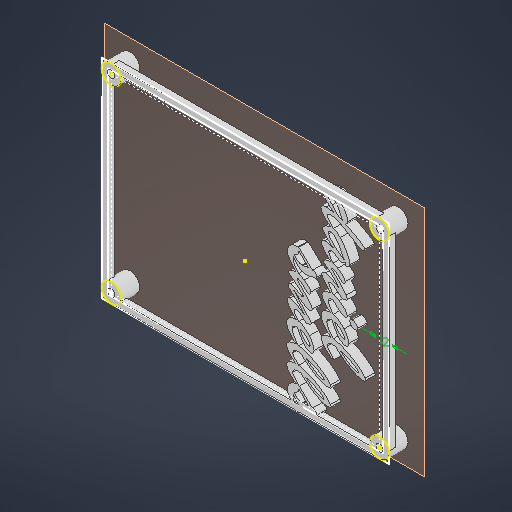
# Autodesk Inventor part: pcb standoff v1
Saved by Autodesk Inventor 2026.1 (Build 301233020, 233B)
## iProperties
Created: 2026-02-25
Part Number: pcb standoff v1
Material: Generic
Document SubType Name: Modeling
Designer: stoof
Density: 1 g/cm^3
Appearance: Default
Author: stoof
Autodesk Inventor part; units mm, degrees
ref_plane "YZ Plane" through (0, 0, 0) normal (1, 0, 0) x (0, 1, 0)
ref_plane "XZ Plane" through (0, 0, 0) normal (0, 1, 0) x (-1, 0, 0)
ref_plane "XY Plane" through (0, 0, 0) normal (0, 0, 1) x (1, 0, 0)
ref_plane "Work Plane1" through (0, 0, 0) normal (0, 0, 1) x (1, 0, 0)
sketch "Sketch1" plane through (0, 0, 0) normal (0, 0, 1) x (1, 0, 0)
  circle A0 centre (42.5, 30) radius 1.05 projected
  circle A1 centre (42.5, -30) radius 1.05 projected
  circle A2 centre (-42.5, -30) radius 1.05 projected
  circle A3 centre (-42.5, 30) radius 1.05 projected
  circle A4 centre (-42.5, 30) radius 3.05
  circle A5 centre (42.5, 30) radius 3.05
  circle A6 centre (42.5, -30) radius 3.05
  circle A7 centre (-42.5, -30) radius 3.05
  point P0 (0, 0)
  dimension "d0" = 2
  dimension "d1" = 2
  dimension "d2" = 2
  dimension "d3" = 2
  constraints: 4 centre point
  measures "d0" radial gap between concentric circles of A3 A4
  measures "d1" radial gap between concentric circles of A0 A5
  measures "d2" radial gap between concentric circles of A1 A6
  measures "d3" radial gap between concentric circles of A2 A7
extrude "Extrusion1" add sketch "Sketch1" along normal blind 6 contours A0 | A1 | A2 | A3 | A4 | A5 | A6 | A7
sketch "Sketch2" plane through (-42.5, 30, 6) normal (0, 0, 1) x (1, 0, 0)
  line L0 (85, 0) -> (0, 0) construction
  line L1 (0, 0) -> (0, -60) construction
  line L2 (0, -60) -> (85, -60) construction
  line L3 (85, -60) -> (85, 0) construction
  line L4 (86, 1) -> (-1, 1)
  line L5 (-1, 1) -> (-1, -61)
  line L6 (-1, -61) -> (86, -61)
  line L7 (86, -61) -> (86, 1)
  line L8 (88, 3) -> (-3, 3)
  line L9 (-3, 3) -> (-3, -63)
  line L10 (-3, -63) -> (88, -63)
  line L11 (88, -63) -> (88, 3)
  circle A0 centre (0, -60) radius 3.05 projected
  circle A1 centre (85, -60) radius 3.05 projected
  circle A2 centre (85, 0) radius 3.05 projected
  circle A3 centre (0, 0) radius 3.05 projected
  point P0 (42.5, -30)
  point P1 (85.55, -63)
  point P2 (88, -60.55)
  point P3 (88, 0.55)
  point P4 (85.55, 3)
  point P5 (-0.55, 3)
  point P6 (-3, 0.55)
  point P7 (-3, -60.55)
  point P8 (-0.55, -63)
  point P9 (88, -0.55)
  point P10 (86, -2.8814)
  point P11 (86, -57.1186)
  point P12 (88, -59.45)
  point P13 (0.55, 3)
  point P14 (2.8814, 1)
  point P15 (82.1186, 1)
  point P16 (84.45, 3)
  point P17 (84.45, -63)
  point P18 (82.1186, -61)
  point P19 (2.8814, -61)
  point P20 (0.55, -63)
  point P21 (-1, -2.8814)
  point P22 (-3, -0.55)
  point P23 (-3, -59.45)
  point P24 (-1, -57.1186)
  dimension "d6" = 1
  dimension "d7" = 2
  constraints: 24 end point, 6 parallel, 3 perpendicular, 1 horizontal, 6 other
  measures "d6" distance between parallel lines of L3 L7
  measures "d7" distance between parallel lines of L7 L11
extrude "Extrusion2" add sketch "Sketch2" against normal blind 2 contours L4 A3 L8 A2 | A2 L11 A1 L7 | A1 L10 A0 L6 | L5 A0 L9 A3
sketch "Sketch3" plane through (0, 0, 6) normal (0, 0, 1) x (1, 0, 0)
  line L0 (38.1473, 32.6739) -> (38.1473, 6.3376) construction
  line L1 (38.1473, 6.3376) -> (30.1508, 6.3376) construction
  line L2 (30.1508, 6.3376) -> (30.1508, 32.6739) construction
  line L3 (30.1508, 32.6739) -> (38.1473, 32.6739) construction
  line L4 (27.1524, 12.2976) -> (27.1524, -13.1616) construction
  line L5 (27.1524, -13.1616) -> (19.2192, -13.1616) construction
  line L6 (19.2192, -13.1616) -> (19.2192, 12.2976) construction
  line L7 (19.2192, 12.2976) -> (27.1524, 12.2976) construction
  line L8 (16.645, 12.1571) -> (16.9259, 12.1571)
  spline S0 degree 2 poles (16.9259, 12.1571) (20.0444, 9.1931) (21.2947, 8.0834) knots 0 0 0 1 1 1
  spline S1 degree 2 poles (21.2947, 8.0834) (22.6994, 7.8305) (22.6994, 6.8753) knots 0 0 0 1 1 1
  spline S2 degree 2 poles (22.6994, 6.8753) (22.6994, 6.6365) (22.5589, 6.3555) knots 0 0 0 1 1 1
  line L9 (22.5589, 6.3555) -> (22.3482, 6.2853)
  spline S3 degree 2 poles (22.3482, 6.2853) (22.2077, 6.3415) (21.9549, 6.3415) knots 0 0 0 1 1 1
  spline S4 degree 2 poles (21.9549, 6.3415) (21.7301, 6.3415) (20.5501, 6.0044) (19.7494, 5.8217) (19.2437, 5.8217) knots 0 0 0 1 2 3 3 3
  spline S5 degree 2 poles (19.2437, 5.8217) (18.4992, 5.8217) (17.1085, 6.5101) (15.8302, 7.8165) (15.17, 8.8419) knots 0 0 0 1 2 3 3 3
  spline S6 degree 2 poles (15.17, 8.8419) (15.0998, 8.4346) (15.0998, 8.1958) knots 0 0 0 1 1 1
  spline S7 degree 2 poles (15.0998, 8.1958) (15.0998, 7.7181) (15.5633, 6.6365) (16.364, 5.4987) (16.9962, 4.7401) knots 0 0 0 1 2 3 3 3
  line L10 (16.9962, 4.7401) -> (16.2235, 4.7401)
  spline S8 degree 2 poles (16.2235, 4.7401) (14.7907, 6.2151) (13.3157, 8.5188) (13.3157, 9.3617) knots 0 0 0 1 2 2 2
  spline S9 degree 2 poles (13.3157, 9.3617) (13.3157, 10.4433) (14.2288, 11.3564) knots 0 0 0 1 1 1
  spline S10 degree 2 poles (14.2288, 11.3564) (14.7767, 11.8902) (15.7881, 12.1571) (16.645, 12.1571) knots 0 0 0 1 2 2 2
  line L11 (18.4009, 7.8867) -> (20.0725, 8.0834)
  spline S11 degree 2 poles (20.0725, 8.0834) (19.2718, 8.7998) (16.9962, 11.1176) knots 0 0 0 1 1 1
  spline S12 degree 2 poles (16.9962, 11.1176) (16.8416, 10.4293) (16.3359, 9.9376) (15.6195, 9.4741) knots 0 0 0 1 2 2 2
  spline S13 degree 2 poles (15.6195, 9.4741) (15.9426, 8.7015) (17.0523, 7.8586) (18.0076, 7.8586) knots 0 0 0 1 2 2 2
  spline S14 degree 2 poles (18.0076, 7.8586) (18.1199, 7.8586) (18.3026, 7.8727) (18.4009, 7.8867) knots 0 0 0 1 2 2 2
  spline S15 degree 2 poles (15.3947, -0.4434) (16.7995, -2.0308) (18.8645, -4.2924) (20.0585, -5.5848) (20.8873, -6.5681) (20.8873, -6.7085) knots 0 0 0 1 2 3 4 4 4
  spline S16 degree 2 poles (20.8873, -6.7085) (20.8873, -6.9754) (19.7775, -7.4531) (19.4544, -7.4531) knots 0 0 0 1 2 2 2
  spline S17 degree 2 poles (19.4544, -7.4531) (19.2297, -7.4531) (17.6142, -5.9921) (16.659, -5.2757) (16.1393, -5.2757) knots 0 0 0 1 2 3 3 3
  spline S18 degree 2 poles (16.1393, -5.2757) (15.8302, -5.2757) (15.4509, -5.6831) (15.4509, -5.9781) knots 0 0 0 1 2 2 2
  spline S19 degree 2 poles (15.4509, -5.9781) (15.4509, -6.3012) (16.1393, -7.2283) (17.0102, -8.2257) knots 0 0 0 1 2 2 2
  line L12 (17.0102, -8.2257) -> (16.2095, -8.2257)
  spline S20 degree 2 poles (16.2095, -8.2257) (15.2683, -7.2423) (13.8917, -5.6128) (13.2174, -4.4048) (13.2174, -4.0114) knots 0 0 0 1 2 3 3 3
  spline S21 degree 2 poles (13.2174, -4.0114) (13.2174, -3.6462) (13.7652, -3.1686) (14.1586, -3.1686) knots 0 0 0 1 2 2 2
  spline S22 degree 2 poles (14.1586, -3.1686) (14.5519, -3.1686) (15.3526, -3.4495) (16.4483, -4.0114) (17.9935, -4.9526) (18.6397, -5.3459) knots 0 0 0 1 2 3 4 4 4
  spline S23 degree 2 poles (18.6397, -5.3459) (17.6845, -4.18) (15.9285, -2.3679) (14.6081, -1.216) (14.2288, -0.8929) knots 0 0 0 1 2 3 3 3
  spline S24 degree 2 poles (14.2288, -0.8929) (13.5124, -0.2467) (13.5124, 0.3011) knots 0 0 0 1 1 1
  spline S25 degree 2 poles (13.5124, 0.3011) (13.5124, 0.8911) (14.3693, 0.8911) knots 0 0 0 1 1 1
  spline S26 degree 2 poles (14.3693, 0.8911) (14.7064, 0.8911) (16.4904, 0.0061) (17.853, -0.8227) knots 0 0 0 1 2 2 2
  spline S27 degree 2 poles (17.853, -0.8227) (17.9514, -0.8929) (18.148, -0.8929) knots 0 0 0 1 1 1
  spline S28 degree 2 poles (18.148, -0.8929) (18.3728, -0.8929) (18.3728, -0.6541) knots 0 0 0 1 1 1
  spline S29 degree 2 poles (18.3728, -0.6541) (18.3728, -0.4153) (17.4176, 0.5399) (15.9145, 1.9025) knots 0 0 0 1 2 2 2
  spline S30 degree 2 poles (15.9145, 1.9025) (15.4931, 2.2818) (14.1305, 3.237) (13.6669, 3.6444) (13.6669, 3.8551) knots 0 0 0 1 2 3 3 3
  spline S31 degree 2 poles (13.6669, 3.8551) (13.6669, 4.2625) (15.1278, 4.9789) (16.1112, 4.9789) knots 0 0 0 1 2 2 2
  spline S32 degree 2 poles (16.1112, 4.9789) (16.8135, 4.9789) (17.853, 4.5153) (18.6116, 4.0237) knots 0 0 0 1 2 2 2
  spline S33 degree 2 poles (18.6116, 4.0237) (19.7213, 3.2511) (20.6766, 2.2677) (20.6766, 1.7339) knots 0 0 0 1 2 2 2
  spline S34 degree 2 poles (20.6766, 1.7339) (20.6766, 1.3968) (20.4097, 0.9332) (20.1849, 0.9332) knots 0 0 0 1 2 2 2
  spline S35 degree 2 poles (20.1849, 0.9332) (19.9461, 0.9332) (18.8364, 1.7761) (18.2604, 2.4223) knots 0 0 0 1 2 2 2
  spline S36 degree 2 poles (18.2604, 2.4223) (17.9233, 2.7735) (16.954, 3.3915) (16.7433, 3.3915) knots 0 0 0 1 2 2 2
  spline S37 degree 2 poles (16.7433, 3.3915) (16.4343, 3.3915) (16.4343, 3.1527) knots 0 0 0 1 1 1
  spline S38 degree 2 poles (16.4343, 3.1527) (16.4343, 2.9561) (18.0357, 1.3687) (19.918, -0.5136) (21.1682, -2.1431) (21.1682, -2.705) knots 0 0 0 1 2 3 4 4 4
  spline S39 degree 2 poles (21.1682, -2.705) (21.1682, -3.0422) (20.6485, -3.4917) (20.2692, -3.4917) knots 0 0 0 1 2 2 2
  spline S40 degree 2 poles (20.2692, -3.4917) (20.0304, -3.4917) (18.7099, -2.8034) (16.7714, -1.4829) (15.3947, -0.4434) knots 0 0 0 1 2 3 3 3
  line L13 (16.5466, -9.9816) -> (16.2657, -9.9816)
  spline S41 degree 2 poles (16.2657, -9.9816) (15.5914, -9.9816) (14.8328, -10.6418) (14.8328, -11.1756) knots 0 0 0 1 2 2 2
  spline S42 degree 2 poles (14.8328, -11.1756) (14.8328, -11.7375) (15.3667, -12.9456) (16.2235, -14.1256) (16.9681, -14.9825) knots 0 0 0 1 2 3 3 3
  line L14 (16.9681, -14.9825) -> (16.2657, -14.9825)
  spline S43 degree 2 poles (16.2657, -14.9825) (14.7064, -13.6901) (13.0488, -11.4285) (13.0488, -10.2625) knots 0 0 0 1 2 2 2
  spline S44 degree 2 poles (13.0488, -10.2625) (13.0488, -9.2511) (14.6362, -8.0571) (15.9988, -8.0571) knots 0 0 0 1 2 2 2
  spline S45 degree 2 poles (15.9988, -8.0571) (17.2069, -8.0571) (19.1735, -9.1809) (20.2551, -10.4452) knots 0 0 0 1 2 2 2
  spline S46 degree 2 poles (20.2551, -10.4452) (20.9997, -11.3161) (21.7582, -13.0299) (21.7582, -13.7042) knots 0 0 0 1 2 2 2
  spline S47 degree 2 poles (21.7582, -13.7042) (21.7582, -14.238) (21.2666, -14.8701) (20.7749, -14.8701) knots 0 0 0 1 2 2 2
  spline S48 degree 2 poles (20.7749, -14.8701) (20.0444, -14.8701) (18.6116, -13.8025) (17.2069, -11.597) (16.5466, -9.9816) knots 0 0 0 1 2 3 3 3
  spline S49 degree 2 poles (17.2911, -10.094) (17.6985, -11.1194) (18.8926, -12.5804) (19.9742, -13.2827) (20.2271, -13.2827) knots 0 0 0 1 2 3 3 3
  spline S50 degree 2 poles (20.2271, -13.2827) (20.494, -13.2827) (20.494, -13.0439) knots 0 0 0 1 1 1
  spline S51 degree 2 poles (20.494, -13.0439) (20.494, -12.8332) (19.9602, -11.9061) (19.1173, -10.9649) (17.9795, -10.2064) (17.2911, -10.094) knots 0 0 0 1 2 3 4 4 4
  line L15 (17.0945, -20.475) -> (16.2516, -20.475)
  spline S52 degree 2 poles (16.2516, -20.475) (13.0769, -18.0729) (13.0769, -16.5698) knots 0 0 0 1 1 1
  spline S53 degree 2 poles (13.0769, -16.5698) (13.0769, -15.7551) (14.8469, -14.8279) (16.2938, -14.8279) knots 0 0 0 1 2 2 2
  spline S54 degree 2 poles (16.2938, -14.8279) (17.4597, -14.8279) (20.6766, -15.9236) (23.9918, -17.7779) (26.4501, -19.7726) (26.9417, -20.6155) knots 0 0 0 1 2 3 4 4 4
  spline S55 degree 2 poles (26.9417, -20.6155) (27.1524, -20.9667) (27.1524, -21.1493) knots 0 0 0 1 1 1
  spline S56 degree 2 poles (27.1524, -21.1493) (27.1524, -21.4021) (26.731, -21.5567) (26.2113, -21.5567) knots 0 0 0 1 2 2 2
  spline S57 degree 2 poles (26.2113, -21.5567) (24.6239, -21.5567) (19.9882, -18.9579) (17.5721, -16.6401) knots 0 0 0 1 2 2 2
  spline S58 degree 2 poles (17.5721, -16.6401) (16.9681, -16.5277) (16.645, -16.5277) knots 0 0 0 1 1 1
  spline S59 degree 2 poles (16.645, -16.5277) (15.9145, -16.5277) (15.0014, -17.1598) (15.0014, -17.7217) knots 0 0 0 1 2 2 2
  spline S60 degree 2 poles (15.0014, -17.7217) (15.0014, -18.0027) (15.4509, -18.6769) (16.1112, -19.4074) (17.0945, -20.475) knots 0 0 0 1 2 3 3 3
  spline S61 degree 2 poles (19.1595, -17.0474) (19.7494, -17.6374) (21.2385, -18.7612) (22.9382, -19.7445) (24.2868, -20.3064) (24.6239, -20.3064) knots 0 0 0 1 2 3 4 4 4
  spline S62 degree 2 poles (24.6239, -20.3064) (24.8908, -20.3064) (24.8908, -20.1238) knots 0 0 0 1 1 1
  spline S63 degree 2 poles (24.8908, -20.1238) (24.8908, -20.0536) (24.7644, -19.8569) knots 0 0 0 1 1 1
  spline S64 degree 2 poles (24.7644, -19.8569) (24.1884, -19.1546) (20.8592, -17.4127) (19.1595, -17.0474) knots 0 0 0 1 2 2 2
  line L16 (17.0945, -25.8411) -> (16.2516, -25.8411)
  spline S65 degree 2 poles (16.2516, -25.8411) (13.0769, -23.439) (13.0769, -21.9359) knots 0 0 0 1 1 1
  spline S66 degree 2 poles (13.0769, -21.9359) (13.0769, -21.1212) (14.8469, -20.1941) (16.2938, -20.1941) knots 0 0 0 1 2 2 2
  spline S67 degree 2 poles (16.2938, -20.1941) (17.4597, -20.1941) (20.6766, -21.2898) (23.9918, -23.144) (26.4501, -25.1387) (26.9417, -25.9816) knots 0 0 0 1 2 3 4 4 4
  spline S68 degree 2 poles (26.9417, -25.9816) (27.1524, -26.3328) (27.1524, -26.5154) knots 0 0 0 1 1 1
  spline S69 degree 2 poles (27.1524, -26.5154) (27.1524, -26.7682) (26.731, -26.9228) (26.2113, -26.9228) knots 0 0 0 1 2 2 2
  spline S70 degree 2 poles (26.2113, -26.9228) (24.6239, -26.9228) (19.9882, -24.324) (17.5721, -22.0062) knots 0 0 0 1 2 2 2
  spline S71 degree 2 poles (17.5721, -22.0062) (16.9681, -21.8938) (16.645, -21.8938) knots 0 0 0 1 1 1
  spline S72 degree 2 poles (16.645, -21.8938) (15.9145, -21.8938) (15.0014, -22.5259) (15.0014, -23.0878) knots 0 0 0 1 2 2 2
  spline S73 degree 2 poles (15.0014, -23.0878) (15.0014, -23.3688) (15.4509, -24.0431) (16.1112, -24.7735) (17.0945, -25.8411) knots 0 0 0 1 2 3 3 3
  spline S74 degree 2 poles (19.1595, -22.4136) (19.7494, -23.0035) (21.2385, -24.1273) (22.9382, -25.1107) (24.2868, -25.6726) (24.6239, -25.6726) knots 0 0 0 1 2 3 4 4 4
  spline S75 degree 2 poles (24.6239, -25.6726) (24.8908, -25.6726) (24.8908, -25.4899) knots 0 0 0 1 1 1
  spline S76 degree 2 poles (24.8908, -25.4899) (24.8908, -25.4197) (24.7644, -25.223) knots 0 0 0 1 1 1
  spline S77 degree 2 poles (24.7644, -25.223) (24.1884, -24.5207) (20.8592, -22.7788) (19.1595, -22.4136) knots 0 0 0 1 2 2 2
  line L17 (16.645, -25.6866) -> (16.9259, -25.6866)
  spline S78 degree 2 poles (16.9259, -25.6866) (20.0444, -28.6506) (21.2947, -29.7603) knots 0 0 0 1 1 1
  spline S79 degree 2 poles (21.2947, -29.7603) (22.6994, -30.0132) (22.6994, -30.9684) knots 0 0 0 1 1 1
  spline S80 degree 2 poles (22.6994, -30.9684) (22.6994, -31.2072) (22.5589, -31.4882) knots 0 0 0 1 1 1
  line L18 (22.5589, -31.4882) -> (22.3482, -31.5584)
  spline S81 degree 2 poles (22.3482, -31.5584) (22.2077, -31.5022) (21.9549, -31.5022) knots 0 0 0 1 1 1
  spline S82 degree 2 poles (21.9549, -31.5022) (21.7301, -31.5022) (20.5501, -31.8394) (19.7494, -32.022) (19.2437, -32.022) knots 0 0 0 1 2 3 3 3
  spline S83 degree 2 poles (19.2437, -32.022) (18.4992, -32.022) (17.1085, -31.3337) (15.8302, -30.0272) (15.17, -29.0018) knots 0 0 0 1 2 3 3 3
  spline S84 degree 2 poles (15.17, -29.0018) (15.0998, -29.4092) (15.0998, -29.648) knots 0 0 0 1 1 1
  spline S85 degree 2 poles (15.0998, -29.648) (15.0998, -30.1256) (15.5633, -31.2072) (16.364, -32.3451) (16.9962, -33.1036) knots 0 0 0 1 2 3 3 3
  line L19 (16.9962, -33.1036) -> (16.2235, -33.1036)
  spline S86 degree 2 poles (16.2235, -33.1036) (14.7907, -31.6287) (13.3157, -29.3249) (13.3157, -28.482) knots 0 0 0 1 2 2 2
  spline S87 degree 2 poles (13.3157, -28.482) (13.3157, -27.4004) (14.2288, -26.4873) knots 0 0 0 1 1 1
  spline S88 degree 2 poles (14.2288, -26.4873) (14.7767, -25.9535) (15.7881, -25.6866) (16.645, -25.6866) knots 0 0 0 1 2 2 2
  line L20 (18.4009, -29.957) -> (20.0725, -29.7603)
  spline S89 degree 2 poles (20.0725, -29.7603) (19.2718, -29.0439) (16.9962, -26.7261) knots 0 0 0 1 1 1
  spline S90 degree 2 poles (16.9962, -26.7261) (16.8416, -27.4144) (16.3359, -27.9061) (15.6195, -28.3697) knots 0 0 0 1 2 2 2
  spline S91 degree 2 poles (15.6195, -28.3697) (15.9426, -29.1423) (17.0523, -29.9851) (18.0076, -29.9851) knots 0 0 0 1 2 2 2
  spline S92 degree 2 poles (18.0076, -29.9851) (18.1199, -29.9851) (18.3026, -29.9711) (18.4009, -29.957) knots 0 0 0 1 2 2 2
  spline S93 degree 2 poles (27.9348, 27.2516) (26.7829, 28.263) (25.1815, 29.8503) (24.3948, 30.8477) (24.3948, 31.0303) knots 0 0 0 1 2 3 3 3
  spline S94 degree 2 poles (24.3948, 31.0303) (24.3948, 31.3394) (25.3641, 32.0839) (26.8531, 32.6036) (27.6117, 32.6036) knots 0 0 0 1 2 3 3 3
  spline S95 degree 2 poles (27.6117, 32.6036) (28.7214, 32.6036) (30.9831, 30.4544) (32.4721, 27.7011) (32.4721, 27.0128) knots 0 0 0 1 2 3 3 3
  spline S96 degree 2 poles (32.4721, 27.0128) (32.4721, 26.4509) (31.7697, 25.9171) knots 0 0 0 1 1 1
  spline S97 degree 2 poles (31.7697, 25.9171) (33.6099, 25.0321) (36.4756, 23.4447) (37.8663, 22.3631) (37.8663, 22.1383) knots 0 0 0 1 2 3 3 3
  spline S98 degree 2 poles (37.8663, 22.1383) (37.8663, 21.8855) (37.3746, 21.464) (37.0656, 21.464) knots 0 0 0 1 2 2 2
  spline S99 degree 2 poles (37.0656, 21.464) (36.4756, 21.464) (33.5678, 23.2059) (30.8145, 24.9057) (28.1455, 26.1137) (27.0217, 26.1137) knots 0 0 0 1 2 3 4 4 4
  spline S100 degree 2 poles (27.0217, 26.1137) (25.9822, 26.1137) (25.9822, 25.4535) knots 0 0 0 1 1 1
  spline S101 degree 2 poles (25.9822, 25.4535) (25.9822, 25.0461) (26.8953, 23.8381) (27.9629, 22.7143) knots 0 0 0 1 2 2 2
  line L21 (27.9629, 22.7143) -> (27.12, 22.7143)
  spline S102 degree 2 poles (27.12, 22.7143) (23.9313, 25.1866) (23.9313, 26.5211) knots 0 0 0 1 1 1
  spline S103 degree 2 poles (23.9313, 26.5211) (23.9313, 27.069) (24.746, 27.5325) (25.5608, 27.5325) knots 0 0 0 1 2 2 2
  spline S104 degree 2 poles (25.5608, 27.5325) (26.6565, 27.5325) (27.9348, 27.2516) knots 0 0 0 1 1 1
  spline S105 degree 2 poles (30.7302, 26.4087) (30.3931, 27.4342) (28.8619, 30.1734) (28.581, 30.4544) knots 0 0 0 1 2 2 2
  spline S106 degree 2 poles (28.581, 30.4544) (28.3422, 30.7072) (27.0919, 31.1006) (26.7689, 31.1006) knots 0 0 0 1 2 2 2
  spline S107 degree 2 poles (26.7689, 31.1006) (26.5722, 31.1006) (26.3193, 30.8758) (26.3193, 30.6932) knots 0 0 0 1 2 2 2
  spline S108 degree 2 poles (26.3193, 30.6932) (26.3193, 30.5387) (26.6003, 30.1313) (27.401, 29.2182) (27.5134, 29.0918) knots 0 0 0 1 2 3 3 3
  spline S109 degree 2 poles (27.5134, 29.0918) (27.6819, 28.8951) (28.8198, 27.5606) (29.4519, 26.9425) (30.2526, 26.5071) (30.7302, 26.4087) knots 0 0 0 1 2 3 4 4 4
  spline S110 degree 2 poles (30.0138, 21.3657) (31.6012, 19.6238) (33.1323, 16.3508) (33.1323, 15.4658) knots 0 0 0 1 2 2 2
  spline S111 degree 2 poles (33.1323, 15.4658) (33.1323, 15.227) (32.725, 14.8056) (32.2052, 14.5668) (32.0788, 14.5668) knots 0 0 0 1 2 3 3 3
  spline S112 degree 2 poles (32.0788, 14.5668) (31.8681, 14.5668) (31.6714, 14.8899) (31.545, 15.2972) knots 0 0 0 1 2 2 2
  spline S113 degree 2 poles (31.545, 15.2972) (31.3624, 15.2129) (30.7864, 14.9601) (30.4212, 14.8196) (30.2948, 14.8196) knots 0 0 0 1 2 3 3 3
  spline S114 degree 2 poles (30.2948, 14.8196) (30.0138, 14.8196) (28.5107, 15.9294) (27.8084, 16.3789) (27.2886, 16.3789) knots 0 0 0 1 2 3 3 3
  spline S115 degree 2 poles (27.2886, 16.3789) (26.4458, 16.3789) (26.4458, 15.6063) knots 0 0 0 1 1 1
  spline S116 degree 2 poles (26.4458, 15.6063) (26.4458, 14.7915) (27.9348, 13.0918) knots 0 0 0 1 1 1
  line L22 (27.9348, 13.0918) -> (27.2465, 13.0918)
  spline S117 degree 2 poles (27.2465, 13.0918) (24.0296, 15.9855) (24.0296, 17.2358) knots 0 0 0 1 1 1
  spline S118 degree 2 poles (24.0296, 17.2358) (24.0296, 17.6853) (24.6056, 18.0646) (25.1815, 18.0646) knots 0 0 0 1 2 2 2
  spline S119 degree 2 poles (25.1815, 18.0646) (26.0805, 18.0646) (27.8084, 17.4043) knots 0 0 0 1 1 1
  spline S120 degree 2 poles (27.8084, 17.4043) (25.9541, 19.076) (24.3808, 20.7055) (24.3808, 21.2393) knots 0 0 0 1 2 2 2
  spline S121 degree 2 poles (24.3808, 21.2393) (24.3808, 21.4921) (25.2517, 22.2366) (26.6424, 22.8266) (27.3869, 22.8266) knots 0 0 0 1 2 3 3 3
  spline S122 degree 2 poles (27.3869, 22.8266) (27.9207, 22.8266) (28.6372, 22.6159) (29.3957, 22.0259) (30.0138, 21.3657) knots 0 0 0 1 2 3 3 3
  spline S123 degree 2 poles (31.2781, 15.8872) (29.9155, 18.8653) (28.005, 21.3938) (27.0077, 21.3938) knots 0 0 0 1 2 2 2
  spline S124 degree 2 poles (27.0077, 21.3938) (26.6284, 21.3938) (26.1648, 21.1409) (26.1648, 20.9302) knots 0 0 0 1 2 2 2
  spline S125 degree 2 poles (26.1648, 20.9302) (26.1648, 20.8038) (26.3193, 20.4807) knots 0 0 0 1 1 1
  spline S126 degree 2 poles (26.3193, 20.4807) (27.0358, 19.2726) (29.3114, 17.2779) (31.2781, 15.8872) knots 0 0 0 1 2 2 2
  spline S127 degree 2 poles (30.0279, 5.464) (27.7803, 7.4869) (26.9093, 7.4869) knots 0 0 0 1 1 1
  spline S128 degree 2 poles (26.9093, 7.4869) (26.4177, 7.4869) (26.4177, 7.0795) knots 0 0 0 1 1 1
  spline S129 degree 2 poles (26.4177, 7.0795) (26.4177, 6.7564) (27.106, 5.6888) (28.005, 4.551) knots 0 0 0 1 2 2 2
  line L23 (28.005, 4.551) -> (27.2184, 4.551)
  spline S130 degree 2 poles (27.2184, 4.551) (25.617, 6.1805) (24.1982, 7.9223) (24.1982, 8.4702) knots 0 0 0 1 2 2 2
  spline S131 degree 2 poles (24.1982, 8.4702) (24.1982, 9.4114) (25.4343, 9.4114) knots 0 0 0 1 1 1
  spline S132 degree 2 poles (25.4343, 9.4114) (25.7996, 9.4114) (26.502, 9.1866) (27.2746, 8.7792) (28.7074, 7.9504) (29.6064, 7.4166) knots 0 0 0 1 2 3 4 4 4
  spline S133 degree 2 poles (29.6064, 7.4166) (29.2693, 8.0769) (28.286, 9.0602) knots 0 0 0 1 1 1
  spline S134 degree 2 poles (28.286, 9.0602) (27.6679, 9.6923) (26.5581, 10.5913) (25.1955, 11.6028) (24.732, 12.0804) (24.732, 12.3192) knots 0 0 0 1 2 3 4 4 4
  spline S135 degree 2 poles (24.732, 12.3192) (24.732, 12.6844) (26.2631, 13.3025) (27.2886, 13.3025) knots 0 0 0 1 2 2 2
  spline S136 degree 2 poles (27.2886, 13.3025) (27.9067, 13.3025) (28.6231, 13.0215) (29.2693, 12.5861) knots 0 0 0 1 2 2 2
  spline S137 degree 2 poles (29.2693, 12.5861) (30.4914, 11.7994) (31.6152, 10.6616) (31.6152, 10.1278) knots 0 0 0 1 2 2 2
  spline S138 degree 2 poles (31.6152, 10.1278) (31.6152, 9.7625) (31.3624, 9.313) (31.1095, 9.313) knots 0 0 0 1 2 2 2
  spline S139 degree 2 poles (31.1095, 9.313) (30.9971, 9.313) (30.7443, 9.4535) (30.5336, 9.6221) (30.2386, 9.903) knots 0 0 0 1 2 3 3 3
  spline S140 degree 2 poles (30.2386, 9.903) (28.2298, 11.7151) (27.6398, 11.7151) knots 0 0 0 1 1 1
  spline S141 degree 2 poles (27.6398, 11.7151) (27.3027, 11.7151) (27.3027, 11.4904) knots 0 0 0 1 1 1
  spline S142 degree 2 poles (27.3027, 11.4904) (27.3027, 11.364) (28.1876, 10.5632) (29.6205, 9.313) (31.1797, 7.6133) (31.8962, 6.5176) knots 0 0 0 1 2 3 4 4 4
  spline S143 degree 2 poles (31.8962, 6.5176) (32.3176, 5.9136) (32.3176, 5.5062) knots 0 0 0 1 1 1
  spline S144 degree 2 poles (32.3176, 5.5062) (32.3176, 5.3236) (31.3062, 4.9724) (30.8005, 4.9724) knots 0 0 0 1 2 2 2
  spline S145 degree 2 poles (30.8005, 4.9724) (30.5476, 4.9724) (30.0279, 5.464) knots 0 0 0 1 1 1
  line L24 (27.9629, -0.8432) -> (27.1341, -0.8432)
  spline S146 degree 2 poles (27.1341, -0.8432) (25.7012, 0.2665) (24.2403, 2.1769) (24.2403, 2.8512) knots 0 0 0 1 2 2 2
  spline S147 degree 2 poles (24.2403, 2.8512) (24.2403, 3.7924) (26.207, 4.7055) (27.3729, 4.7055) knots 0 0 0 1 2 2 2
  spline S148 degree 2 poles (27.3729, 4.7055) (27.8224, 4.7055) (28.6372, 4.5229) (29.171, 4.27) (29.7188, 3.9329) knots 0 0 0 1 2 3 3 3
  spline S149 degree 2 poles (29.7188, 3.9329) (32.2614, 2.3034) (32.2614, 0.9548) knots 0 0 0 1 1 1
  spline S150 degree 2 poles (32.2614, 0.9548) (32.2614, 0.2665) (31.7276, 0.2665) knots 0 0 0 1 1 1
  spline S151 degree 2 poles (31.7276, 0.2665) (31.3483, 0.2665) (29.789, 1.1655) (29.466, 1.5167) knots 0 0 0 1 2 2 2
  spline S152 degree 2 poles (29.466, 1.5167) (28.4967, 2.5141) (27.7522, 3.1181) (27.2605, 3.1181) knots 0 0 0 1 2 2 2
  spline S153 degree 2 poles (27.2605, 3.1181) (26.8531, 3.1181) (26.3053, 2.5) (26.3053, 2.0084) knots 0 0 0 1 2 2 2
  spline S154 degree 2 poles (26.3053, 2.0084) (26.3053, 1.4746) (27.0919, 0.1822) (27.9629, -0.8432) knots 0 0 0 1 2 2 2
  spline S155 degree 2 poles (33.0761, -0.0706) (33.0761, 0.2103) (33.5116, 0.7301) (33.8487, 0.7301) knots 0 0 0 1 2 2 2
  spline S156 degree 2 poles (33.8487, 0.7301) (34.3545, 0.7301) (35.5906, -0.2252) (35.5906, -0.7449) knots 0 0 0 1 2 2 2
  spline S157 degree 2 poles (35.5906, -0.7449) (35.5906, -1.0821) (35.1692, -1.5456) (34.7618, -1.5456) knots 0 0 0 1 2 2 2
  spline S158 degree 2 poles (34.7618, -1.5456) (34.2702, -1.5456) (33.0761, -0.6044) (33.0761, -0.0706) knots 0 0 0 1 2 2 2
  line L25 (27.5415, -2.5851) -> (27.2605, -2.5851)
  spline S159 degree 2 poles (27.2605, -2.5851) (26.5862, -2.5851) (25.8277, -3.2454) (25.8277, -3.7792) knots 0 0 0 1 2 2 2
  spline S160 degree 2 poles (25.8277, -3.7792) (25.8277, -4.3411) (26.3615, -5.5491) (27.2184, -6.7291) (27.9629, -7.586) knots 0 0 0 1 2 3 3 3
  line L26 (27.9629, -7.586) -> (27.2605, -7.586)
  spline S161 degree 2 poles (27.2605, -7.586) (25.7012, -6.2936) (24.0437, -4.032) (24.0437, -2.8661) knots 0 0 0 1 2 2 2
  spline S162 degree 2 poles (24.0437, -2.8661) (24.0437, -1.8547) (25.631, -0.6606) (26.9936, -0.6606) knots 0 0 0 1 2 2 2
  spline S163 degree 2 poles (26.9936, -0.6606) (28.2017, -0.6606) (30.1683, -1.7844) (31.25, -3.0487) knots 0 0 0 1 2 2 2
  spline S164 degree 2 poles (31.25, -3.0487) (31.9945, -3.9196) (32.753, -5.6334) (32.753, -6.3077) knots 0 0 0 1 2 2 2
  spline S165 degree 2 poles (32.753, -6.3077) (32.753, -6.8415) (32.2614, -7.4736) (31.7697, -7.4736) knots 0 0 0 1 2 2 2
  spline S166 degree 2 poles (31.7697, -7.4736) (31.0393, -7.4736) (29.6064, -6.406) (28.2017, -4.2006) (27.5415, -2.5851) knots 0 0 0 1 2 3 3 3
  spline S167 degree 2 poles (28.286, -2.6975) (28.6933, -3.723) (29.8874, -5.1839) (30.969, -5.8863) (31.2219, -5.8863) knots 0 0 0 1 2 3 3 3
  spline S168 degree 2 poles (31.2219, -5.8863) (31.4888, -5.8863) (31.4888, -5.6475) knots 0 0 0 1 1 1
  spline S169 degree 2 poles (31.4888, -5.6475) (31.4888, -5.4368) (30.955, -4.5096) (30.1121, -3.5684) (28.9743, -2.8099) (28.286, -2.6975) knots 0 0 0 1 2 3 4 4 4
  line L27 (28.0893, -13.0785) -> (27.2465, -13.0785)
  spline S170 degree 2 poles (27.2465, -13.0785) (24.0717, -10.6764) (24.0717, -9.1734) knots 0 0 0 1 1 1
  spline S171 degree 2 poles (24.0717, -9.1734) (24.0717, -8.3586) (25.8417, -7.4315) (27.2886, -7.4315) knots 0 0 0 1 2 2 2
  spline S172 degree 2 poles (27.2886, -7.4315) (28.4545, -7.4315) (31.6714, -8.5272) (34.9866, -10.3814) (37.4449, -12.3762) (37.9365, -13.219) knots 0 0 0 1 2 3 4 4 4
  spline S173 degree 2 poles (37.9365, -13.219) (38.1473, -13.5702) (38.1473, -13.7528) knots 0 0 0 1 1 1
  spline S174 degree 2 poles (38.1473, -13.7528) (38.1473, -14.0057) (37.7258, -14.1602) (37.2061, -14.1602) knots 0 0 0 1 2 2 2
  spline S175 degree 2 poles (37.2061, -14.1602) (35.6187, -14.1602) (30.9831, -11.5614) (28.5669, -9.2436) knots 0 0 0 1 2 2 2
  spline S176 degree 2 poles (28.5669, -9.2436) (27.9629, -9.1312) (27.6398, -9.1312) knots 0 0 0 1 1 1
  spline S177 degree 2 poles (27.6398, -9.1312) (26.9093, -9.1312) (25.9962, -9.7634) (25.9962, -10.3253) knots 0 0 0 1 2 2 2
  spline S178 degree 2 poles (25.9962, -10.3253) (25.9962, -10.6062) (26.4458, -11.2805) (27.106, -12.0109) (28.0893, -13.0785) knots 0 0 0 1 2 3 3 3
  spline S179 degree 2 poles (30.1543, -9.651) (30.7443, -10.241) (32.2333, -11.3648) (33.933, -12.3481) (35.2816, -12.91) (35.6187, -12.91) knots 0 0 0 1 2 3 4 4 4
  spline S180 degree 2 poles (35.6187, -12.91) (35.8856, -12.91) (35.8856, -12.7274) knots 0 0 0 1 1 1
  spline S181 degree 2 poles (35.8856, -12.7274) (35.8856, -12.6571) (35.7592, -12.4605) knots 0 0 0 1 1 1
  spline S182 degree 2 poles (35.7592, -12.4605) (35.1833, -11.7581) (31.854, -10.0162) (30.1543, -9.651) knots 0 0 0 1 2 2 2
  point P0 (0, 0)
  dimension "d3" = 2
  constraints: 4 other
extrude "Extrusion3" add sketch "Sketch3" against normal blind 3
hole "Hole1" at (-42.5, 30, 6) at (42.5, 30, 6) at (42.5, -30, 6) at (-42.5, -30, 6) direction (0, 0, -1) diameter 2.3 end through all
body "Solid1"
